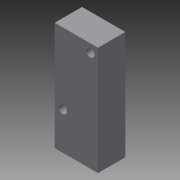
# Autodesk Inventor part: Limit Switch
Saved by Autodesk Inventor 2013 (Build 170138000, 138)
## iProperties
Created: 2013-03-16
Part Number: Limit Switch
Material: Generic
Document SubType Name: Modeling
Designer: Arpan
Density: 1 g/cm^3
Author: Arpan
Autodesk Inventor part; units mm, degrees
ref_plane "YZ Plane" through (0, 0, 0) normal (1, 0, 0) x (0, 1, 0)
ref_plane "XZ Plane" through (0, 0, 0) normal (0, 1, 0) x (-1, 0, 0)
ref_plane "XY Plane" through (0, 0, 0) normal (0, 0, 1) x (1, 0, 0)
sketch "Sketch1" plane through (0, 0, 0) normal (0, 0, 1) x (1, 0, 0)
  line L0 (0, 0) -> (0, 28.7274)
  line L1 (0, 28.7274) -> (15.8242, 28.7274)
  line L2 (15.8242, 28.7274) -> (15.8242, 0)
  line L3 (15.8242, 0) -> (0, 0)
  circle A0 centre (12.9667, 25.8699) radius 1.5875
  circle A1 centre (12.9667, 25.8699) radius 2.8575
  circle A2 centre (2.8575, 2.8575) radius 1.5875
  circle A3 centre (2.8575, 2.8575) radius 2.8575
  dimension "d0" = 28.7274
  dimension "d1" = 15.8242
  dimension "d2" = 3.175
  dimension "d3" = 5.715
  dimension "d4" = 3.175
  dimension "d5" = 5.715
  constraints: 8 end point, 4 centre point, 4 tangent, 2 coincident, 2 parallel, 1 perpendicular, 1 vertical
  measures "d0" distance of L0.start L0.end
  measures "d1" distance of L0.end L1.end
  measures "d2" diameter of A0
  measures "d3" diameter of A1
  measures "d4" diameter of A2
  measures "d5" diameter of A3
extrude "Extrusion1" add sketch "Sketch1" along normal blind 10.0076
sketch "Sketch2" plane through (0, 0, 10.0076) normal (0, 0, 1) x (1, 0, 0)
  line L0 (0, 0) -> (15.8242, 0) projected
  line L1 (15.8242, 28.7274) -> (0, 28.7274) projected
  line L2 (0, 0) -> (0, -10.9982)
  line L3 (0, -10.9982) -> (15.8242, -10.9982)
  line L4 (15.8242, -10.9982) -> (15.8242, 0)
  dimension "d8" = 10.9982
  constraints: 6 end point, 2 perpendicular, 1 parallel
  measures "d8" distance of L0.start L2.end
extrude "Extrusion2" add sketch "Sketch2" against normal blind 10.0076
body "Solid1"
